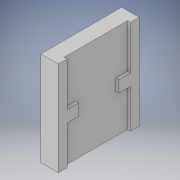
# Autodesk Inventor part: BlockBase
Saved by Autodesk Inventor 2019 (Build 230136000, 136)
## iProperties
Created: 2020-01-25
Part Number: BlockBase
Material: Generic
Document SubType Name: Modeling
Designer: james
Density: 1 g/cm^3
Appearance: Default
Author: james
Autodesk Inventor part; units mm, degrees
ref_plane "YZ Plane" through (0, 0, 0) normal (1, 0, 0) x (0, 1, 0)
ref_plane "XZ Plane" through (0, 0, 0) normal (0, 1, 0) x (-1, 0, 0)
ref_plane "XY Plane" through (0, 0, 0) normal (0, 0, 1) x (1, 0, 0)
sketch "Sketch1" plane through (0, 0, 0) normal (1, 0, 0) x (0, 1, 0)
  line L0 (482.3395, 530.3412) -> (-338.3345, 530.3412)
  line L1 (-338.3345, 530.3412) -> (-338.3345, -174.5088)
  line L2 (-338.3345, -174.5088) -> (482.3395, -174.5088)
  line L3 (482.3395, -174.5088) -> (482.3395, 530.3412)
  point P0 (0, 0)
  dimension "d0" = 820.674
  dimension "d1" = 704.85
  constraints: 8 end point, 2 parallel, 1 horizontal, 1 perpendicular
  measures "d0" distance of L0.start L0.end
  measures "d1" distance of L0.end L1.end
extrude "Extrusion1" add sketch "Sketch1" along normal blind 127
sketch "Sketch2" plane through (127, 0, 0) normal (1, 0, 0) x (0, 0, -1)
  line L0 (174.5088, 482.3395) -> (-530.3412, 482.3395) projected
  line L1 (-530.3412, -338.3345) -> (174.5088, -338.3345) projected
  line L2 (-530.3412, 482.3395) -> (-454.1412, 482.3395)
  line L3 (-454.1412, 482.3395) -> (-454.1412, -338.3345)
  line L4 (-454.1412, -338.3345) -> (-530.3412, -338.3345)
  line L5 (-530.3412, -338.3345) -> (-530.3412, 482.3395)
  line L6 (174.5088, 482.3395) -> (98.3088, 482.3395)
  line L7 (98.3088, 482.3395) -> (98.3088, -338.3345)
  line L8 (98.3088, -338.3345) -> (174.5088, -338.3345)
  line L9 (174.5088, -338.3345) -> (174.5088, 482.3395)
  line L10 (174.5088, -338.3345) -> (174.5088, 482.3395) projected
  point P0 (0, 0)
  dimension "d4" = 76.2
  dimension "d5" = 76.2
  dimension "d6" = 0
  constraints: 16 end point, 4 parallel, 3 point on line, 2 horizontal, 2 perpendicular
  measures "d4" distance between parallel lines of L5 L3
  measures "d5" distance between parallel lines of L9 L7
  measures "d6" distance between parallel lines of L10 L9
extrude "Extrusion2" add sketch "Sketch2" along normal blind 25.4 contours L9 L1 L7 L0 | L3 L1 L5 L0
sketch "Sketch3" plane through (127, 0, 0) normal (1, 0, 0) x (0, 0, -1)
  line L0 (-454.1412, 482.3395) -> (-454.1412, -338.3345) projected
  line L1 (-352.5412, 101.3395) -> (-454.1412, 101.3395)
  line L2 (-454.1412, 101.3395) -> (-454.1412, -0.2605)
  line L3 (-454.1412, -0.2605) -> (-352.5412, -0.2605)
  line L4 (-352.5412, -0.2605) -> (-352.5412, 101.3395)
  line L5 (98.3088, -338.3345) -> (98.3088, 482.3395) projected
  line L6 (-3.2912, 101.3395) -> (98.3088, 101.3395)
  line L7 (98.3088, 101.3395) -> (98.3088, -0.2605)
  line L8 (98.3088, -0.2605) -> (-3.2912, -0.2605)
  line L9 (-3.2912, -0.2605) -> (-3.2912, 101.3395)
  line L10 (98.3088, 482.3395) -> (-454.1412, 482.3395) projected
  point P0 (0, 0)
  dimension "d9" = 101.6
  dimension "d10" = 101.6
  dimension "d11" = 101.6
  dimension "d12" = 101.6
  dimension "d13" = 381
  constraints: 16 end point, 4 parallel, 3 point on line, 2 horizontal, 2 perpendicular
  measures "d9" distance of L6.start L6.end
  measures "d10" distance of L8.end L6.start
  measures "d11" distance of L3.end L1.start
  measures "d12" distance of L1.start L1.end
  measures "d13" distance between parallel lines of L10 L1
extrude "Extrusion3" add sketch "Sketch3" along normal blind 25.4
body "Solid1"
